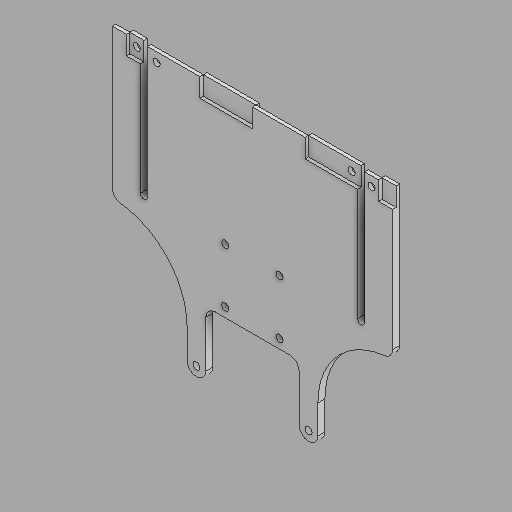
# Autodesk Inventor part: RC_CAR_BASE_PLATE
Saved by Autodesk Inventor 2025.2 (Build 292293000, 293)
## iProperties
Created: 2025-10-26
Part Number: RC_CAR_BASE_PLATE
Material: Generic
Document SubType Name: Modeling
Designer: Ben
Density: 1 g/cm^3
Appearance: Default
Author: Ben
Autodesk Inventor part; units mm, degrees
ref_plane "YZ Plane" through (0, 0, 0) normal (1, 0, 0) x (0, 1, 0)
ref_plane "XZ Plane" through (0, 0, 0) normal (0, 1, 0) x (-1, 0, 0)
ref_plane "XY Plane" through (0, 0, 0) normal (0, 0, 1) x (1, 0, 0)
sketch "Sketch1" plane through (0, 0, 0) normal (0, 0, 1) x (1, 0, 0)
  line L0 (-133.35, 0) -> (133.35, 0) projected
  line L1 (0, -231.14) -> (0, 231.14) projected
  line L2 (-44.45, -165.1) -> (44.45, 165.1) construction
  line L3 (44.45, -165.1) -> (-44.45, 165.1) construction
  line L4 (-95.25, -88.9) -> (-44.45, -88.9)
  line L5 (-44.45, 88.9) -> (-95.25, 88.9)
  line L6 (-95.25, 88.9) -> (-95.25, -88.9)
  line L7 (-95.25, -88.9) -> (-44.45, 88.9) construction
  line L8 (-44.45, -88.9) -> (-95.25, 88.9) construction
  line L9 (95.25, -88.9) -> (44.45, -88.9)
  line L10 (44.45, 88.9) -> (95.25, 88.9)
  line L11 (95.25, 88.9) -> (95.25, -88.9)
  line L12 (95.25, -88.9) -> (44.45, 88.9) construction
  line L13 (44.45, -88.9) -> (95.25, 88.9) construction
  line L14 (44.45, -165.1) -> (44.45, -88.9)
  line L15 (44.45, 88.9) -> (44.45, 165.1)
  line L16 (-44.45, 165.1) -> (-44.45, 88.9)
  line L17 (-44.45, -88.9) -> (-44.45, -165.1)
  line L18 (-31.75, 120.65) -> (31.75, 120.65)
  line L19 (31.75, 120.65) -> (31.75, 165.1)
  line L20 (-31.75, 165.1) -> (-31.75, 120.65)
  line L21 (-31.75, 120.65) -> (31.75, 165.1) construction
  line L22 (31.75, 120.65) -> (-31.75, 165.1) construction
  line L23 (-31.75, -120.65) -> (31.75, -120.65)
  line L24 (31.75, -120.65) -> (31.75, -165.1)
  line L25 (-31.75, -165.1) -> (-31.75, -120.65)
  line L26 (-31.75, -120.65) -> (31.75, -165.1) construction
  line L27 (31.75, -120.65) -> (-31.75, -165.1) construction
  line L28 (44.45, 165.1) -> (31.75, 165.1)
  line L29 (-31.75, 165.1) -> (-44.45, 165.1)
  line L30 (-44.45, -165.1) -> (-31.75, -165.1)
  line L31 (31.75, -165.1) -> (44.45, -165.1)
  point P0 (0, 0)
  point P1 (-69.85, 0)
  point P2 (69.85, 0)
  point P3 (0, 142.875)
  point P4 (0, -142.875)
  dimension "d0" = 88.9
  dimension "d1" = 330.2
  dimension "d3" = 50.8
  dimension "d4" = 12.7
  dimension "d5" = 44.45
  dimension "d27" = 76.2
  constraints: 60 end point, 12 parallel, 10 midpoint, 6 horizontal, 6 perpendicular, 4 point on line, 4 other
  measures "d0" distance of L2.end L3.end
  measures "d1" distance of L3.end L2.start
  measures "d3" distance of L4.start L4.end
  measures "d4" distance between parallel lines of L16 L20
  measures "d5" distance of L20.start L18.start
  measures "d27" distance between parallel lines of L29 L5
extrude "Extrusion1" add sketch "Sketch1" along normal blind 4.7625
sketch "Sketch2" plane through (0, 0, 4.7625) normal (0, 0, 1) x (1, 0, 0)
  line L0 (0, -231.14) -> (0, 231.14) projected
  line L1 (-133.35, 0) -> (133.35, 0) projected
  line L2 (31.75, -165.1) -> (44.45, -165.1) projected
  line L3 (44.45, -165.1) -> (44.45, -88.9) projected
  line L4 (-31.75, -120.65) -> (31.75, -120.65) projected
  point P0 (0, 0)
  point P1 (38.1, -158.75)
  point P2 (-38.1, -158.75)
  point P3 (38.1, 158.75)
  point P4 (-38.1, 158.75)
  point P5 (18.5, -114.3)
  point P6 (-18.5, -114.3)
  point P7 (-18.5, -77.3)
  point P8 (18.5, -77.3)
  point P9 (18.5, 77.3)
  point P10 (-18.5, 77.3)
  point P11 (18.5, 114.3)
  point P12 (-18.5, 114.3)
  dimension "d10" = 6.35
  dimension "d11" = 6.35
  dimension "d12" = 37
  dimension "d13" = 37
  dimension "d14" = 6.35
  constraints: 8 symmetric about line, 2 horizontal alignment, 2 vertical alignment
  measures "d10" distance from line of L2 point (38.1, -158.75)
  measures "d11" distance from line of L3 point (38.1, -158.75)
  measures "d12" distance of point (-18.5, -114.3) point (18.5, -114.3)
  measures "d13" distance of point (18.5, -77.3) point (18.5, -114.3)
  measures "d14" distance from line of L4 point (18.5, -114.3)
hole "Hole1" at (38.1, -158.75, 4.7625) at (-38.1, -158.75, 4.7625) at (38.1, 158.75, 4.7625) at (-38.1, 158.75, 4.7625) at (18.5, -114.3, 4.7625) at (-18.5, -114.3, 4.7625) at (-18.5, -77.3, 4.7625) at (18.5, -77.3, 4.7625) at (18.5, 77.3, 4.7625) at (-18.5, 77.3, 4.7625) at (18.5, 114.3, 4.7625) at (-18.5, 114.3, 4.7625) direction (0, 0, -1) diameter 4.7625 end through all
sketch "Sketch3" plane through (0, 0, 4.7625) normal (0, 0, 1) x (1, 0, 0)
  line L0 (73.8188, -76.2) -> (73.8187, 76.2) construction
  line L1 (76.2, -76.2) -> (76.2, 76.2)
  line L2 (71.4375, 76.2) -> (71.4375, -76.2)
  arc A0 (71.4375, -76.2) -> (76.2, -76.2) centre (73.8188, -76.2) ccw
  arc A1 (76.2, 76.2) -> (71.4375, 76.2) centre (73.8187, 76.2) ccw
  line L3 (-73.8188, -76.2) -> (-73.8188, 76.2) construction
  line L4 (-71.4375, -76.2) -> (-71.4375, 76.2)
  line L5 (-76.2, 76.2) -> (-76.2, -76.2)
  arc A2 (-76.2, -76.2) -> (-71.4375, -76.2) centre (-73.8188, -76.2) ccw
  arc A3 (-71.4375, 76.2) -> (-76.2, 76.2) centre (-73.8188, 76.2) ccw
  line L6 (0, -231.14) -> (0, 231.14) projected
  line L7 (-133.35, 0) -> (133.35, 0) projected
  line L8 (95.25, -88.9) -> (95.25, 88.9) projected
  point P0 (0, 0)
  point P1 (73.8187, 0)
  point P2 (-73.8187, 0)
  dimension "d22" = 152.4
  dimension "d23" = 4.7625
  dimension "d24" = 19.05
  constraints: 16 end point, 8 point on circle, 8 tangent, 4 centre point, 2 horizontal alignment, 2 midpoint, 2 parallel, 2 vertical, 3 other
  measures "d22" distance of L0.end L0.start
  measures "d23" distance between parallel lines of L1 L2
  measures "d24" distance between parallel lines of L8 L1
extrude "Extrusion2" cut sketch "Sketch3" along normal through all both and the other way through all
fillet "Fillet1" radius 6.35 16 edges at (44.45, 165.1, 2.3813) (31.75, 165.1, 2.3813) (95.25, 88.9, 2.3813) (31.75, 120.65, 2.3813) (-31.75, 120.65, 2.3813) (-31.75, 165.1, 2.3813) (-44.45, 165.1, 2.3813) (-95.25, 88.9, 2.3813) (-95.25, -88.9, 2.3813) (-44.45, -165.1, 2.3813) (-31.75, -165.1, 2.3813) (-31.75, -120.65, 2.3813) (31.75, -120.65, 2.3813) (31.75, -165.1, 2.3813) (44.45, -165.1, 2.3813) (95.25, -88.9, 2.3813)
fillet "Fillet2" radius 50.8 4 edges at (44.45, -88.9, 2.3813) (-44.45, -88.9, 2.3813) (-44.45, 88.9, 2.3813) (44.45, 88.9, 2.3813)
sketch "Sketch4" plane through (0, 0, 4.7625) normal (0, 0, 1) x (1, 0, 0)
  line L0 (-133.35, 0) -> (133.35, 0) projected
  line L1 (0, -231.14) -> (0, 231.14) projected
  line L2 (95.25, -82.55) -> (95.25, 82.55) projected
  line L3 (95.25, 12.7) -> (-95.25, 12.7)
  line L4 (-95.25, 12.7) -> (-95.25, 165.1)
  line L5 (-95.25, 165.1) -> (95.25, 165.1)
  line L6 (95.25, 165.1) -> (95.25, 12.7)
  arc A0 (-31.75, 158.75) -> (-44.45, 158.75) centre (-38.1, 158.75) ccw projected
  point P0 (0, 0)
  point P1 (-95.25, 82.55)
  dimension "d30" = 12.7
  constraints: 8 end point, 2 parallel, 1 horizontal, 1 perpendicular, 1 point on line, 1 tangent, 1 vertical alignment
  measures "d30" distance between parallel lines of L0 L3
extrude "Extrusion3" cut sketch "Sketch4" along normal through all both and the other way through all contours L3 L4 L5 L1 | L1 L5 L6 L2 L3
sketch "Sketch5" plane through (0, 0, 4.7625) normal (0, 0, 1) x (1, 0, 0)
  line L0 (-95.25, 12.7) -> (-76.2, 12.7) projected
  line L1 (-76.2, 12.7) -> (-85.725, 12.7)
  line L2 (-85.725, 12.7) -> (-85.725, 0)
  line L3 (-85.725, 0) -> (-76.2, 0)
  line L4 (-76.2, 0) -> (-76.2, 12.7)
  line L5 (71.4375, 12.7) -> (-71.4375, 12.7) projected
  line L6 (0, 0) -> (-35.7188, 0)
  line L7 (-35.7188, 0) -> (-35.7187, 12.7)
  line L8 (-35.7187, 12.7) -> (0, 12.7)
  line L9 (0, 12.7) -> (0, 0)
  line L10 (71.4375, 12.7) -> (35.7188, 12.7)
  line L11 (35.7188, 12.7) -> (35.7188, 0)
  line L12 (35.7188, 0) -> (71.4375, 0)
  line L13 (71.4375, 0) -> (71.4375, 12.7)
  line L14 (95.25, -82.55) -> (95.25, 12.7) projected
  line L15 (95.25, 12.7) -> (85.725, 12.7)
  line L16 (85.725, 12.7) -> (85.725, 0)
  line L17 (85.725, 0) -> (95.25, 0)
  line L18 (95.25, 0) -> (95.25, 12.7)
  line L19 (95.25, 12.7) -> (76.2, 12.7) projected
  point P0 (-85.725, 12.7)
  dimension "d33" = 35.7188
  dimension "d34" = 35.7188
  constraints: 32 end point, 8 parallel, 4 horizontal, 4 perpendicular, 3 horizontal alignment, 2 midpoint, 1 coincident, 1 point on line, 1 vertical alignment
  measures "d33" distance of L6.start L6.end
  measures "d34" distance of L11.end L12.end
extrude "Extrusion4" cut sketch "Sketch5" against normal blind 2.3813
sketch "Sketch6" plane through (0, 0, 0) normal (0, 0, -1) x (-1, 0, 0)
  line L0 (95.25, 12.7) -> (95.25, -82.55) projected
  line L1 (85.725, 0) -> (95.25, 0)
  line L2 (95.25, 0) -> (95.25, 12.7)
  line L3 (95.25, 12.7) -> (85.725, 12.7)
  line L4 (85.725, 12.7) -> (85.725, 0)
  line L5 (71.4375, 12.7) -> (-71.4375, 12.7) projected
  line L6 (35.7188, 0) -> (71.4375, 0)
  line L7 (71.4375, 0) -> (71.4375, 12.7)
  line L8 (71.4375, 12.7) -> (35.7188, 12.7)
  line L9 (35.7188, 12.7) -> (35.7188, 0)
  line L10 (0, 0) -> (35.7188, 0) projected
  line L11 (0, 0) -> (-35.7188, 0)
  line L12 (-35.7188, 0) -> (-35.7188, 12.7)
  line L13 (-35.7188, 12.7) -> (0, 12.7)
  line L14 (0, 12.7) -> (0, 0)
  line L15 (-85.725, 0) -> (-85.725, 12.7) projected
  line L16 (-76.2, 12.7) -> (-76.2, -76.2) projected
  line L17 (-85.725, 0) -> (-76.2, 0)
  line L18 (-76.2, 0) -> (-76.2, 12.7)
  line L19 (-76.2, 12.7) -> (-85.725, 12.7)
  line L20 (-85.725, 12.7) -> (-85.725, 0)
  constraints: 32 end point, 8 parallel, 4 horizontal, 4 perpendicular, 1 collinear, 1 point on line
extrude "Extrusion5" cut sketch "Sketch6" against normal blind 2.3813 contours L0 L1 L4 L3 | L7 L6 L9 L5 | L14 L11 L12 L5 | L15 L19 L16 L17
sketch "Sketch7" plane through (0, 0, 0) normal (0, 0, -1) x (-1, 0, 0)
  line L0 (71.4375, 12.7) -> (71.4375, 0) projected
  line L1 (0, -200.66) -> (0, 48.26) projected
  line L2 (-35.7188, 12.7) -> (-71.4375, 12.7) projected
  line L3 (-85.725, 0) -> (-85.725, 12.7) projected
  point P0 (0, 0)
  point P1 (80.9625, 6.35)
  point P2 (65.0875, 6.35)
  point P3 (-80.9625, 6.35)
  point P4 (-65.0875, 6.35)
  dimension "d39" = 6.35
  dimension "d40" = 6.35
  dimension "d41" = 4.7625
  constraints: 3 horizontal alignment, 2 symmetric about line
  measures "d39" distance from line of L0 point (65.088, 6.35)
  measures "d40" distance from line of L2 point (-65.088, 6.35)
  measures "d41" distance from line of L3 point (-80.963, 6.35)
hole "Hole2" at (-80.9625, 6.35, 0) at (-65.0875, 6.35, 0) at (80.9625, 6.35, 0) at (65.0875, 6.35, 0) direction (0, 0, 1) diameter 4.7625 end through all
body "Solid1"
